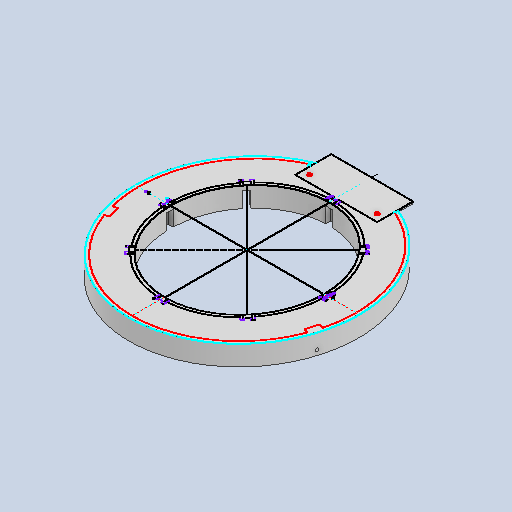
# Autodesk Inventor part: capacete_2
Saved by Autodesk Inventor 2024.3 (Build 283343000, 343)
## iProperties
Created: 2024-07-08
Part Number: capacete_2
Material: Genérico
Document SubType Name: Modeling
Designer: lostv
Density: 1 g/cm^3
Appearance: Padrão
Author: lostv
Autodesk Inventor part; units mm, degrees
ref_plane "YZ Plane" through (0, 0, 0) normal (1, 0, 0) x (0, 1, 0)
ref_plane "XZ Plane" through (0, 0, 0) normal (0, 1, 0) x (-1, 0, 0)
ref_plane "XY Plane" through (0, 0, 0) normal (0, 0, 1) x (1, 0, 0)
sketch "Esboço1" plane through (0, 0, 0) normal (0, 1, 0) x (-1, 0, 0)
  ellipse E0 centre (0, 0) end of major axis (75, 0) minor radius 80.5 (75, 0) -> (0, 80.5) ccw
  line L0 (0, 80.5) -> (0, 0)
  line L1 (0, 0) -> (75, 0)
  line L2 (0, 0) -> (54.8745, 54.8745)
  line L3 (0, 0) -> (77.6042, 0) construction
  line L4 (75, 0) -> (78, 0)
  ellipse E1 centre (0, 0) end of major axis (0, 83.5) minor radius 78 (53.7651, 60.4941) -> (5, 83.3283) ccw
  ellipse E2 centre (0, 0) end of major axis (0, 83.5) minor radius 78 (77.86, 5) -> (60.3196, 52.9395) ccw
  ellipse E3 centre (0, 0) end of major axis (-75, 0) minor radius 80.5 (0, 80.5) -> (-75, 0) ccw
  line L5 (0, 0) -> (-75, 0)
  line L6 (0, 0) -> (-54.8745, 54.8745)
  line L7 (0, 0) -> (-75, 0) construction
  line L8 (-79.224, 3) -> (-74.9479, 3)
  ellipse E4 centre (0, 0) end of major axis (0, 83.5) minor radius 78 (-5, 83.3283) -> (-53.7651, 60.4941) ccw
  ellipse E5 centre (0, 0) end of major axis (0, 83.5) minor radius 78 (-60.3196, 52.9395) -> (-77.86, 5) ccw
  line L9 (75, 0) -> (-75, 0)
  ellipse E6 centre (0, 0) end of major axis (75, 0) minor radius 80.5 (0, -80.5) -> (75, 0) ccw
  line L10 (0, -80.5) -> (0, 0)
  line L11 (3, -84.7178) -> (3, -80.4356)
  line L12 (5, -84.7178) -> (5, -80.3209)
  line L13 (3, -80.4356) -> (3, -84.7178)
  line L14 (0, 0) -> (54.8745, -54.8745)
  ellipse E7 centre (0, 0) end of major axis (0, -83.5) minor radius 78 (5, -83.3283) -> (53.7651, -60.4941) ccw
  ellipse E8 centre (0, 0) end of major axis (0, -83.5) minor radius 78 (60.3196, -52.9395) -> (77.86, -5) ccw
  line L15 (0, 0) -> (-54.8745, -54.8745)
  ellipse E9 centre (0, 0) end of major axis (-75, 0) minor radius 80.5 (-75, 0) -> (0, -80.5) ccw
  line L16 (-52.9206, -57.0425) -> (-56.079, -59.8863)
  line L17 (-56.8499, -52.5066) -> (-60.0938, -55.4274)
  line L18 (-56.8499, -52.5066) -> (-60.0938, -55.4274)
  line L19 (-52.9206, -57.0425) -> (-56.079, -59.8863)
  line L20 (-3, -84.7178) -> (-3, -80.4356)
  line L21 (-5, -84.7178) -> (-5, -80.3209)
  line L22 (-3, -80.4356) -> (-3, -84.7178)
  ellipse E10 centre (0, 0) end of major axis (0, -83.5) minor radius 78 (-53.7651, -60.4941) -> (-5, -83.3283) ccw
  ellipse E11 centre (0, 0) end of major axis (0, -83.5) minor radius 78 (-77.86, -5) -> (-60.3196, -52.9395) ccw
  line L23 (-79.224, -3) -> (-74.9769, -3)
  line L24 (40, -122.0178) -> (-40, -122.0178)
  line L25 (-40, -122.0178) -> (-40, -122.0178)
  line L26 (0, -122.0178) -> (0, -128.5198) construction
  line L27 (-79.224, -5) -> (-74.8552, -5)
  line L28 (-79.224, 5) -> (-74.8552, 5)
  line L29 (-79.224, -5) -> (-81.524, -5) construction
  line L30 (-81.524, -5) -> (-81.524, -2.5) construction
  line L31 (-81.524, -2.5) -> (-79.224, -2.5) construction
  line L32 (-79.224, -5) -> (-81.524, -5)
  line L33 (-81.524, -2.5) -> (-81.524, -5)
  line L34 (-81.524, -2.5) -> (-79.224, -2.5)
  line L35 (-79.224, -2.5) -> (-79.224, -3)
  line L36 (-79.224, 3) -> (-79.224, 2.5)
  line L37 (-81.524, 2.5) -> (-79.224, 2.5)
  line L38 (-81.524, 2.5) -> (-81.524, 5)
  line L39 (-81.524, 5) -> (-79.224, 5)
  line L40 (-79.224, -3) -> (-79.224, -2.5) construction
  line L41 (-79.224, 2.5) -> (-79.224, 3) construction
  line L42 (-79.224, -2.5) -> (-79.224, 2.5)
  line L43 (-56.079, -59.8863) -> (-60.0938, -55.4274) construction
  line L44 (-61.432, -53.9411) -> (-58.0841, -50.9266)
  line L45 (-54.7407, -61.3726) -> (-51.5348, -58.4859)
  line L46 (-54.7407, -61.3726) -> (-56.45, -62.9116)
  line L47 (-56.45, -62.9116) -> (-58.1228, -61.0537)
  line L48 (-58.1228, -61.0537) -> (-56.4136, -59.5147)
  line L49 (-56.079, -59.8863) -> (-56.4136, -59.5147)
  line L50 (-60.0938, -55.4274) -> (-56.4136, -59.5147)
  line L51 (-61.432, -53.9411) -> (-63.1413, -55.4801)
  line L52 (-63.1413, -55.4801) -> (-61.4684, -57.338)
  line L53 (-61.4684, -57.338) -> (-59.7592, -55.799)
  line L54 (3, -84.7178) -> (-3, -84.7178) construction
  line L55 (-5, -84.7178) -> (-5, -87.0178)
  line L56 (-5, -87.0178) -> (-2.5, -87.0178)
  line L57 (-2.5, -87.0178) -> (-2.5, -84.7178)
  line L58 (-3, -84.7178) -> (-2.5, -84.7178)
  line L59 (5, -84.7178) -> (5, -87.0178)
  line L60 (5, -87.0178) -> (2.5, -87.0178)
  line L61 (2.5, -87.0178) -> (2.5, -84.7178)
  line L62 (3, -84.7178) -> (2.5, -84.7178)
  line L63 (-2.5, -84.7178) -> (2.5, -84.7178)
  line L64 (52.9206, -57.0425) -> (56.079, -59.8863)
  line L65 (56.8499, -52.5066) -> (60.0938, -55.4274)
  line L66 (56.079, -59.8863) -> (60.0938, -55.4274) construction
  line L67 (61.432, -53.9411) -> (58.0841, -50.9266)
  line L68 (54.7407, -61.3726) -> (51.5348, -58.4859)
  line L69 (54.7407, -61.3726) -> (56.45, -62.9116)
  line L70 (56.45, -62.9116) -> (58.1228, -61.0537)
  line L71 (58.1228, -61.0537) -> (56.4136, -59.5147)
  line L72 (56.079, -59.8863) -> (56.4136, -59.5147)
  line L73 (60.0938, -55.4274) -> (56.4136, -59.5147)
  line L74 (61.432, -53.9411) -> (63.1413, -55.4801)
  line L75 (63.1413, -55.4801) -> (61.4684, -57.338)
  line L76 (61.4684, -57.338) -> (59.7592, -55.799)
  line L77 (79.224, 3) -> (74.9479, 3)
  line L78 (79.224, -3) -> (74.9769, -3)
  line L79 (79.224, -5) -> (74.8552, -5)
  line L80 (79.224, 5) -> (74.8552, 5)
  line L81 (79.224, -5) -> (81.524, -5)
  line L82 (81.524, -5) -> (81.524, -2.5)
  line L83 (81.524, -2.5) -> (79.224, -2.5)
  line L84 (79.224, -2.5) -> (79.224, -3)
  line L85 (79.224, 3) -> (79.224, 2.5)
  line L86 (81.524, 2.5) -> (79.224, 2.5)
  line L87 (81.524, 2.5) -> (81.524, 5)
  line L88 (81.524, 5) -> (79.224, 5)
  line L89 (79.224, -2.5) -> (79.224, 2.5)
  line L90 (63.1413, 55.4801) -> (61.4684, 57.338)
  line L91 (61.432, 53.9411) -> (63.1413, 55.4801)
  line L92 (61.4684, 57.338) -> (59.7592, 55.799)
  line L93 (56.8499, 52.5066) -> (60.0938, 55.4274)
  line L94 (61.432, 53.9411) -> (58.0841, 50.9266)
  line L95 (60.0938, 55.4274) -> (56.4136, 59.5147)
  line L96 (56.079, 59.8863) -> (60.0938, 55.4274) construction
  line L97 (52.9206, 57.0425) -> (56.079, 59.8863)
  line L98 (56.079, 59.8863) -> (56.4136, 59.5147)
  line L99 (58.1228, 61.0537) -> (56.4136, 59.5147)
  line L100 (56.45, 62.9116) -> (58.1228, 61.0537)
  line L101 (54.7407, 61.3726) -> (56.45, 62.9116)
  line L102 (54.7407, 61.3726) -> (51.5348, 58.4859)
  line L103 (-56.079, 59.8863) -> (-56.4136, 59.5147)
  line L104 (-54.7407, 61.3726) -> (-56.45, 62.9116)
  line L105 (-56.45, 62.9116) -> (-58.1228, 61.0537)
  line L106 (-58.1228, 61.0537) -> (-56.4136, 59.5147)
  line L107 (-60.0938, 55.4274) -> (-56.4136, 59.5147)
  line L108 (-61.4684, 57.338) -> (-59.7592, 55.799)
  line L109 (-63.1413, 55.4801) -> (-61.4684, 57.338)
  line L110 (-61.432, 53.9411) -> (-63.1413, 55.4801)
  line L111 (-61.432, 53.9411) -> (-58.0841, 50.9266)
  line L112 (-56.8499, 52.5066) -> (-60.0938, 55.4274)
  line L113 (-52.9206, 57.0425) -> (-56.079, 59.8863)
  line L114 (-54.7407, 61.3726) -> (-51.5348, 58.4859)
  line L115 (3, 84.7178) -> (3, 80.4356)
  line L116 (5, 84.7178) -> (5, 80.3209)
  line L117 (-3, 84.7178) -> (-3, 80.4356)
  line L118 (-5, 84.7178) -> (-5, 80.3209)
  line L119 (3, 84.7178) -> (-3, 84.7178) construction
  line L120 (-5, 84.7178) -> (-5, 87.0178)
  line L121 (-5, 87.0178) -> (-2.5, 87.0178)
  line L122 (-2.5, 87.0178) -> (-2.5, 84.7178)
  line L123 (-3, 84.7178) -> (-2.5, 84.7178)
  line L124 (5, 84.7178) -> (5, 87.0178)
  line L125 (5, 87.0178) -> (2.5, 87.0178)
  line L126 (2.5, 87.0178) -> (2.5, 84.7178)
  line L127 (3, 84.7178) -> (2.5, 84.7178)
  line L128 (-2.5, 84.7178) -> (2.5, 84.7178)
  line L129 (74.9769, -3) -> (74.9479, -3)
  line L130 (-74.9769, -3) -> (-74.9479, -3)
  line L131 (-40, -122.0178) -> (40, -122.0178)
  line L132 (40, -122.0178) -> (40, -87.0178)
  line L133 (-40, -87.0178) -> (-40, -122.0178)
  line L134 (0, 0) -> (0, 112) construction
  line L135 (0, 0) -> (106.5, 0) construction
  line L136 (0, 0) -> (0, -108.5) construction
  line L137 (0, 0) -> (-106.5, 0) construction
  line L138 (0, 0) -> (109.5, 0) construction
  line L139 (0, 0) -> (-109.5, 0) construction
  line L140 (0, 0) -> (0, 115) construction
  line L141 (0, 0) -> (0, -111.5) construction
  line L142 (2.5, -87.0178) -> (2.5, -84.7178)
  line L143 (-2.5, -84.7178) -> (-2.5, -87.0178)
  line L144 (-2.5, -84.7178) -> (2.5, -84.7178)
  line L145 (40, -87.0178) -> (2.5, -87.0178)
  line L146 (-2.5, -87.0178) -> (-40, -87.0178)
  ellipse E12 centre (0, 0) end of major axis (109.5, 0) minor radius 115 (40, -107.0525) -> (-40, -107.0525) ccw
  line L147 (98.3879, 27.868) -> (95.2767, 39.2563)
  line L148 (95.2767, 39.2563) -> (99.3422, 40.3669)
  line L149 (98.3879, 27.868) -> (102.8461, 29.0859)
  line L150 (-98.3879, 27.868) -> (-95.2767, 39.2563)
  line L151 (-95.2767, 39.2563) -> (-99.3422, 40.3669)
  line L152 (-98.3879, 27.868) -> (-102.8461, 29.0859)
  ellipse E13 centre (0, 0) end of major axis (106.5, 0) minor radius 112 (40, -103.8002) -> (102.8461, 29.0859) ccw
  ellipse E14 centre (0, 0) end of major axis (106.5, 0) minor radius 112 (99.3422, 40.3669) -> (-99.3422, 40.3669) ccw
  ellipse E15 centre (0, 0) end of major axis (106.5, 0) minor radius 112 (-102.8461, 29.0859) -> (-40, -103.8002) ccw
  circle A0 centre (33, -94.0178) radius 1.75
  circle A1 centre (-33, -94.0178) radius 1.75
  point P0 (95, 0)
  point P1 (98, 0)
  point P2 (-83.9624, 0)
  point P3 (-55.5336, -59.3952)
  point P4 (-74.9479, -3)
  point P5 (-58.1466, -61.748)
  point P6 (-60.0938, -55.4274)
  point P7 (0, -80.5)
  point P8 (-80.374, -2.5)
  point P9 (-80.374, -5)
  point P10 (-79.224, -2.75)
  point P11 (-79.224, 2.75)
  point P12 (-80.374, 5)
  point P13 (-77.0396, 5)
  point P14 (-55.5954, -62.1421)
  point P15 (-60.6138, -56.5685)
  point P16 (-62.3049, -56.409)
  point P17 (2.5, -85.8678)
  point P18 (-2.75, -84.7178)
  point P19 (3, -82.5767)
  point P20 (79.224, -2.75)
  point P21 (-5, 83.3283)
  point P22 (77.86, -5)
  point P23 (-79.224, 0)
  point P24 (-41.4333, -103.43)
  point P25 (41.4333, -103.43)
  point P26 (40, -101.0029)
  point P27 (3.75, 87.0178)
  point P28 (81.524, -3.75)
  dimension "d46" = 83.5
  dimension "d47" = 78
  dimension "d0" = 75
  dimension "d1" = 80.5
  dimension "d6" = 45
  dimension "d75" = 2.5
  dimension "d76" = 2
  dimension "d78" = 2.3
  dimension "d79" = 2.3
  dimension "d81" = 2
  dimension "d82" = 2.5
  dimension "d83" = 6.6688
  dimension "d85" = 2.5
  dimension "d86" = 2.5
  dimension "d88" = 2.3
  dimension "d91" = 2.5
  dimension "d92" = 2.5
  dimension "d93" = 2.3
  dimension "d94" = 4.2822
  dimension "d95" = 6
  dimension "d109" = 112
  dimension "d110" = 106.5
  dimension "d112" = 106.5
  dimension "d113" = 109.5
  dimension "d114" = 109.5
  dimension "d115" = 115
  dimension "d123" = 24.9822
  dimension "d124" = 24.9761
  dimension "d125" = 80
  dimension "d126" = 40
  dimension "d144" = 35
  dimension "d145" = 3.5
  dimension "d146" = 7
  dimension "d147" = 7
  constraints: 306 end point, 100 symmetric about line, 47 point on line, 21 perpendicular, 17 horizontal, 16 midpoint, 15 coincident, 12 collinear, 12 vertical, 4 parallel, 2 centre point, 1 equal length, 105 other
  measures "d0" distance of L0.end L1.end
  measures "d1" distance of L0.start L0.end
  measures "d6" angle of L3 L2
  measures "d75" distance of point (-80.374, -2.5) point (-80.374, -5)
  measures "d76" distance between parallel lines of L27 L23
  measures "d78" distance from line of point (-79.224, -2.75) L33
  measures "d79" distance from line of point (-79.224, 2.75) L38
  measures "d81" distance from line of L8 point (-77.04, 5)
  measures "d82" distance from line of point (-80.374, 5) L37
  measures "d83" distance of L27.end L29.end
  measures "d85" distance from line of point (-55.595, -62.142) L48
  measures "d86" distance from line of point (-60.614, -56.568) L51
  measures "d88" distance between parallel lines of L43 L52
  measures "d91" distance between parallel lines of L57 L55
  measures "d92" distance from line of L59 point (2.5, -85.868)
  measures "d93" distance from line of point (-2.75, -84.718) L56
  measures "d94" distance of L20.start L20.end
  measures "d95" distance from line of point (3, -82.577) L20
  measures "d109" distance of L15.start L134.end
  measures "d110" distance of L15.start L135.end
  measures "d112" distance of L15.start L137.end
  measures "d113" distance of L138.start L138.end
  measures "d114" distance of L138.start L139.end
  measures "d115" distance of L138.start L140.end
  measures "d123" vertical distance of point (3.75, 87.018) L134.end
  measures "d124" horizontal distance of point (81.524, -3.75) L135.end
  measures "d125" distance between parallel lines of L132 L133
  measures "d126" distance between parallel lines of L136 L132
  measures "d144" distance of L133.start L25.end
  measures "d145" diameter of A0
  measures "d146" distance from line of L132 A0.centre
  measures "d147" distance from line of L145 A0.centre
extrude "Extrusão8" add sketch "Esboço1" against normal blind 20 contours E0 L94 E2 L80 | L79 E8 L67 E6 | L116 E1 L102 E0 | E3 L114 E4 L118 | L28 E5 L111 E3 | E9 L44 E11 L27 | E6 L68 E7 L12 | L21 E10 L45 E9
extrude "Extrusão9" add sketch "Esboço1" against normal blind 20 contours E0 L80 L88 L87 L86 L85 L77 | L129 L78 L84 L83 L82 L81 L79 E6 | E0 L93 L95 L92 L90 L91 L94 | L115 L127 L126 L125 L124 L116 E0 | E3 L118 L120 L121 L122 L123 L117 | E0 L102 L101 L100 L99 L98 L97 | L8 L36 L37 L38 L39 L28 E3 | E9 L27 L32 L33 L34 L35 L23 L130 | L113 L103 L106 L105 L104 L114 E3 | E3 L111 L110 L109 L108 L107 L112 | E6 L12 L59 L60 L61 L62 L11 | L20 L58 L57 L56 L55 L21 E9 | L64 L72 L71 L70 L69 L68 E6 | E6 L67 L74 L75 L76 L73 L65 | L17 L50 L53 L52 L51 L44 E9 | E9 L45 L46 L47 L48 L49 L16
extrude "Extrusão10" add sketch "Esboço1" against normal blind 5 contours E0 L77 L85 L89 L84 L78 L129 E6 | E3 L117 L123 L128 L127 L115 E0 | E0 L97 L98 L95 L93 | E9 L130 L23 L35 L42 L36 L8 E3 | E3 L112 L107 L103 L113 | E6 L11 L62 L63 L58 L20 E9 | E6 L65 L73 L72 L64 | E9 L16 L49 L50 L17
extrude "Extrusão14" add sketch "Esboço1" against normal blind 5 contours E2 L94 L91 L90 L92 L95 L99 L100 L101 L102 E1 L116 L124 L125 L126 L128 L122 L121 L120 L118 E4 L114 L104 L105 L106 L107 L108 L109 L110 L111 E5 L28 L39 L38 L37 L42 L34 L33 L32 L27 E11 L44 L51 L52 L53 L50 L48 L47 L46 L45 E10 L21 L55 L146 L133 E15 L152 L150 L151 E14 L148 L147 L149 E13 L132 L145 L59 L12 E7 L68 L69 L70 L71 L73 L76 L75 L74 L67 E8 L79 L81 L82 L83 L89 L86 L87 L88 L80
extrude "Extrusão15" add sketch "Esboço1" against normal blind 20 contours E13 L149 L147 L148 E14 L151 L150 L152 E15 L133 E12 L132
sketch "Esboço2" plane through (-95.2767, -20, 39.2563) normal (0.9647, 0, -0.2635) x (-0.2635, 0, -0.9647)
  circle A0 centre (5.9, 5) radius 1.75
  line L0 (11.8057, 0) -> (0, 0) projected
  line L1 (11.8057, 15) -> (11.8057, 0) projected
  line L2 (0, 15) -> (0, 0) projected
  point P0 (12.7606, 20)
  dimension "d131" = 3.5
  dimension "d132" = 5
  dimension "d133" = 11.8057
  dimension "d134" = 5.9
  constraints: 1 centre point
  measures "d131" diameter of A0
  measures "d132" distance from line of L0 A0.centre
  measures "d133" distance between parallel lines of L1 L2
  measures "d134" distance from line of L2 A0.centre
extrude "Extrusão16" cut sketch "Esboço2" against normal blind 100
sketch "Esboço3" plane through (98.3879, -20, 27.868) normal (-0.9647, 0, -0.2635) x (-0.2635, 0, 0.9647)
  circle A0 centre (5.9057, 5) radius 1.5
  line L0 (11.8057, 0) -> (0, 0) projected
  line L1 (11.8057, 15) -> (11.8057, 0) projected
  point P0 (-0.9549, 20)
  dimension "d137" = 3
  dimension "d138" = 5
  dimension "d139" = 5.9
  constraints: 1 centre point
  measures "d137" diameter of A0
  measures "d138" distance from line of L0 A0.centre
  measures "d139" distance from line of L1 A0.centre
extrude "Extrusão17" cut sketch "Esboço3" against normal blind 100
extrude "Extrusão18" add sketch "Esboço1" against normal blind 2.5 contours L61 L60 L145 L132 L24 L133 L146 L56 L57 L63
